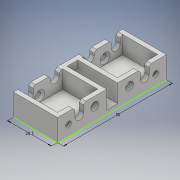
# Autodesk Inventor part: digit_holder_B_no_hole
Saved by Autodesk Inventor 2018 (Build 220112000, 112)
## iProperties
Created: 2021-04-22
Part Number: digit_holder_B_no_hole
Material: Generic
Document SubType Name: Modeling
Designer: Kevin
Density: 1 g/cm^3
Appearance: Default
Author: Kevin
Autodesk Inventor part; units mm, degrees
ref_plane "YZ Plane" through (0, 0, 0) normal (1, 0, 0) x (0, 1, 0)
ref_plane "XZ Plane" through (0, 0, 0) normal (0, 1, 0) x (-1, 0, 0)
ref_plane "XY Plane" through (0, 0, 0) normal (0, 0, 1) x (1, 0, 0)
sketch "Sketch3" plane through (0, 0, 0) normal (0, 0, 1) x (1, 0, 0)
  line L0 (-10.1, 25) -> (10.1, 25)
  line L1 (10.1, 25) -> (10.1, -25)
  line L2 (10.1, -25) -> (-10.1, -25)
  line L3 (-10.1, -25) -> (-10.1, 25)
  point P0 (0, 0)
  dimension "d26" = 20.2
  dimension "d27" = 50
  constraints: 8 end point, 2 parallel, 1 horizontal, 1 perpendicular
  measures "d26" distance of L1.end L2.end
  measures "d27" distance of L0.end L1.end
extrude "Extrusion3" add sketch "Sketch3" along normal blind 1.8
sketch "Sketch4" plane through (0, 0, 1.8) normal (0, 0, 1) x (1, 0, 0)
  line L0 (-8.1, 23) -> (8.1, 23)
  line L1 (8.1, -23) -> (-8.1, -23)
  line L2 (-8.1, 0) -> (-8.1, 2.5)
  line L3 (-8.1, 2.5) -> (8.1, 2.5)
  line L4 (8.1, 4.5) -> (-8.1, 4.5)
  line L5 (-8.1, 0) -> (-8.1, -2.5)
  line L6 (-8.1, -2.5) -> (8.1, -2.5)
  line L7 (8.1, -4.5) -> (-8.1, -4.5)
  line L8 (-8.1, 4.5) -> (-8.1, 23)
  line L9 (8.1, 23) -> (8.1, 4.5)
  line L10 (8.1, 2.5) -> (8.1, -2.5)
  line L11 (8.1, -4.5) -> (8.1, -23)
  line L12 (-10.1, 25) -> (-10.1, -25) projected
  line L13 (10.1, -25) -> (10.1, 25) projected
  line L14 (-10.1, 25) -> (10.1, 25)
  line L15 (10.1, 25) -> (10.1, -25)
  line L16 (10.1, -25) -> (-10.1, -25)
  line L17 (-10.1, -25) -> (-10.1, 25)
  line L18 (-8.1, -23) -> (-8.1, -4.5)
  line L19 (-8.1, -2.5) -> (-8.1, 2.5)
  point P0 (0, 0)
  dimension "d39" = 2.5
  dimension "d40" = 2.5
  dimension "d44" = 2
  dimension "d45" = 2
  dimension "d48" = 2
  dimension "d49" = 2
  dimension "d50" = 2
  dimension "d51" = 2
  dimension "d52" = 2
  dimension "d53" = 2
  dimension "d56" = 2
  dimension "d57" = 2
  constraints: 36 end point, 14 parallel, 4 horizontal, 4 perpendicular, 1 midpoint
  measures "d39" distance from line of point (0, 0) L3
  measures "d40" distance from line of point (0, 0) L6
  measures "d44" distance between parallel lines of L3 L4
  measures "d45" distance between parallel lines of L7 L6
  measures "d48" distance between parallel lines of L14 L0
  measures "d49" distance between parallel lines of L12 L8
  measures "d50" distance between parallel lines of L13 L9
  measures "d51" distance between parallel lines of L17 L18
  measures "d52" distance between parallel lines of L13 L11
  measures "d53" distance between parallel lines of L16 L1
  measures "d56" distance between parallel lines of L12 L2
  measures "d57" distance between parallel lines of L15 L10
extrude "Extrusion4" add sketch "Sketch4" along normal blind 8.2
sketch "Sketch5" plane through (10.1, -25, 0) normal (1, 0, 0) x (0, 0, -1)
  line L0 (-1.8, 27.5) -> (-10, 27.5) projected
  line L1 (-1.8, 22.5) -> (-10, 22.5) projected
  line L2 (-10, 27.5) -> (-1.8, 27.5)
  line L3 (-1.8, 27.5) -> (-1.8, 22.5)
  line L4 (-1.8, 22.5) -> (-10, 22.5)
  line L5 (-10, 22.5) -> (-10, 27.5)
  point P0 (0, 25)
  constraints: 8 end point, 2 parallel, 1 horizontal, 1 perpendicular
extrude "Extrusion5" cut sketch "Sketch5" against normal blind 8.2
sketch "Sketch6" plane through (-10.1, -25, 0) normal (-1, 0, 0) x (0, 0, 1)
  line L0 (1.8, 27.5) -> (1.8, 22.5) projected
  line L1 (1.8, 22.5) -> (6.8, 22.5)
  line L2 (6.8, 22.5) -> (6.8, 27.5)
  line L3 (6.8, 27.5) -> (1.8, 27.5)
  line L4 (1.8, 27.5) -> (1.8, 22.5)
  point P0 (0, 25)
  dimension "d60" = 5
  dimension "d61" = 5
  constraints: 8 end point, 2 parallel, 1 horizontal, 1 perpendicular
  measures "d60" distance of L3.end L2.end
  measures "d61" distance of L2.end L1.end
extrude "Extrusion6" cut sketch "Sketch6" against normal blind 8.2
sketch "Sketch7" plane through (-10.1, -25, 0) normal (-1, 0, 0) x (0, 0, 1)
  line L0 (0, 50) -> (10, 50) projected
  line L1 (0, 0) -> (0, 50) projected
  line L2 (0, 25) -> (10, 25)
  line L3 (0, 0) -> (10, 0)
  circle A0 centre (6.8, 45) radius 2
  circle A1 centre (8, 33) radius 2
  circle A2 centre (8, 17) radius 2
  circle A3 centre (6.8, 5) radius 2
  line L4 (6.8, 7) -> (10, 7)
  line L5 (6.8, 3) -> (10, 3)
  line L6 (10, 50) -> (10, 0) projected
  line L7 (10, 7) -> (10, 3)
  line L8 (6.8, 47) -> (10, 47)
  line L9 (10, 47) -> (10, 43)
  line L10 (10, 43) -> (6.8, 43)
  line L11 (10, 29.5) -> (10, 48) projected
  line L12 (8, 35) -> (10, 35)
  line L13 (10, 35) -> (10, 31)
  line L14 (10, 31) -> (8, 31)
  line L15 (8, 31) -> (8, 35)
  line L16 (10, 20.5) -> (10, 2) projected
  line L17 (8, 19) -> (10, 19)
  line L18 (10, 19) -> (10, 15)
  line L19 (10, 15) -> (8, 15)
  line L20 (8, 15) -> (8, 19)
  point P0 (4.5, 40)
  point P1 (4.5, 10)
  dimension "d66" = 10
  dimension "d67" = 4.5
  dimension "d70" = 5
  dimension "d71" = 6.8
  dimension "d74" = 17
  dimension "d75" = 8
  dimension "d90" = 4
  dimension "d91" = 4
  constraints: 32 end point, 5 horizontal, 4 coincident, 4 parallel, 4 perpendicular, 4 point on circle, 4 symmetric about line, 2 centre point, 2 point on line, 2 tangent, 2 vertical alignment, 6 other
  measures "d66" distance from line of L0 point (4.5, 40)
  measures "d67" distance from line of L1 point (4.5, 40)
  measures "d70" distance from line of L0 point (6.8, 45)
  measures "d71" distance from line of L1 point (6.8, 45)
  measures "d74" distance from line of L0 point (8, 33)
  measures "d75" distance from line of L1 point (8, 33)
  measures "d90" diameter of A0
  measures "d91" diameter of A3
hole "Hole1" at (-10.1, 15, 4.5) at (-10.1, -15, 4.5) direction (1, 0, 0) diameter 2.6 depth 2 tip angle 118
extrude "Extrusion7" cut sketch "Sketch7" against normal blind 2 contours L6 L10 A0 L8 | A0 | L14 A1 L6 | L6 A2 L17 | L6 A1 L12 | L5 A3 L4 L6 | A1 L15 | A1 L15 | A2 L20 | L6 L19 A2 | L20 A2 | A3
sketch "Sketch8" plane through (10.1, -25, 0) normal (1, 0, 0) x (0, 0, -1)
  line L0 (0, 50) -> (-10, 50) projected
  circle A0 centre (-6, 40) radius 2
  circle A1 centre (-6, 10) radius 2
  line L1 (-10, 15) -> (-10, 7) projected
  line L2 (-6, 12) -> (-10, 12)
  line L3 (-10, 12) -> (-10, 8)
  line L4 (-10, 8) -> (-6, 8)
  line L5 (-6, 8) -> (-6, 12)
  line L6 (-10, 43) -> (-10, 35) projected
  line L7 (-6, 42) -> (-10, 42)
  line L8 (-10, 42) -> (-10, 38)
  line L9 (-10, 38) -> (-6, 38)
  line L10 (-6, 38) -> (-6, 42)
  point P0 (0, 25)
  point P1 (-4.8, 45)
  point P2 (-6, 33)
  point P3 (-4.8, 5)
  point P4 (-6, 17)
  dimension "d113" = 4
  dimension "d114" = 4
  constraints: 16 end point, 4 parallel, 3 point on line, 2 coincident, 2 horizontal, 2 perpendicular, 2 vertical alignment, 4 other
hole "Hole3" at (10.1, 20, 4.8) at (10.1, -20, 4.8) direction (-1, 0, 0) diameter 2.6 depth 2 tip angle 118
hole "Hole4" at (10.1, 8, 6) at (10.1, -8, 6) direction (-1, 0, 0) diameter 3.6 depth 2 tip angle 118
extrude "Extrusion8" cut sketch "Sketch8" against normal blind 2
chamfer "Chamfer1" distance 1 angle 45 12 edges at (-9.1, 22, 10) (-9.1, 18, 10) (-9.1, 10, 10) (-9.1, 6, 10) (-9.1, -6, 10) (-9.1, -10, 10) (-9.1, -18, 10) (-9.1, -22, 10) (9.1, -17, 10) (9.1, -13, 10) (9.1, 13, 10) (9.1, 17, 10)
chamfer "Chamfer3" distance 1 angle 45 4 edges at (8.1, 20, 6.1) (8.1, -20, 6.1) (-8.1, -15, 3.2) (-8.1, 15, 3.2)
body "Solid2"
